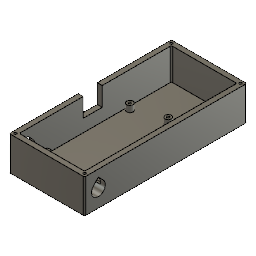
full (Autodesk Fusion 360 design; units mm, degrees)
Autodesk Fusion 360 part; units mm, degrees
sketch "Sketch2" plane through (0, 0, 0) normal (0, 1, 0) x (1, 0, 0)
  line L0 (25, -35.5) -> (-25, -35.5)
  line L1 (-25, -35.5) -> (-25, 35.5)
  line L2 (-25, 35.5) -> (25, 35.5)
  line L3 (25, 35.5) -> (25, -35.5)
  line L4 (25, -35.5) -> (-25, 35.5) construction
  line L5 (-25, -35.5) -> (25, 35.5) construction
  circle A0 centre (-23, -33.5) radius 1
  circle A1 centre (23, -33.5) radius 1
  circle A2 centre (-23, 32.5) radius 1
  circle A3 centre (23, 32.5) radius 1
  line L6 (-25, -1.5) -> (-15, -1.5)
  line L7 (-15, -1.5) -> (-15, 13.5)
  line L8 (-15, 13.5) -> (-25, 13.5)
  line L9 (-25, 13.5) -> (-25, -1.5)
  line L10 (25, 67.5) -> (-21, 67.5)
  line L11 (-21, 67.5) -> (-21, 41.5)
  line L12 (-21, 41.5) -> (25, 41.5)
  line L13 (25, 41.5) -> (25, 67.5)
  line L14 (25, -51.5) -> (7, -51.5)
  line L15 (7, -51.5) -> (7, -41.5)
  line L16 (7, -41.5) -> (25, -41.5)
  line L17 (25, -41.5) -> (25, -51.5)
  line L18 (0, 0) -> (0, -35.5) construction
  line L19 (-25, -41.5) -> (-25, -51.5)
  line L20 (-25, -51.5) -> (-7, -51.5)
  line L21 (-7, -41.5) -> (-25, -41.5)
  line L22 (-7, -51.5) -> (-7, -41.5)
  dimension "d15" = 71
  dimension "d16" = 50
  dimension "d17" = 2
  dimension "d18" = 2
  dimension "d19" = 46
  dimension "d20" = 2
  dimension "d21" = 2
  dimension "d22" = 2
  dimension "d23" = 2
  dimension "d24" = 46
  dimension "d25" = 66
  dimension "d35" = 15
  dimension "d36" = 10
  dimension "d37" = 34
  dimension "d40" = 46
  dimension "d41" = 26
  dimension "d42" = 6
  dimension "d43" = 18
  dimension "d44" = 10
  dimension "d45" = 6
  measures "d17" diameter of A0
  measures "d18" diameter of A1
  measures "d22" diameter of A2
  measures "d37" distance of L0 L6
  measures "d42" distance of L2 L12
  measures "d43" distance of L18.start
  measures "d45" distance of L0 L16
extrude "Extrude2" add sketch "Sketch2" along normal blind 2 contours L0 L1 L2 L3 L6 L7 L8 | L1 L6 L7 L8 L9 makes body 1
extrude "Extrude5" add sketch "Sketch2" along normal blind 18 contours L1 L6 L7 L8 L9 bodies 1
extrude "Extrude7" add sketch "Sketch2" along normal blind 17 separate body contours L10 L11 L12 L13 makes body 2
sketch "Sketch6" plane through (0, 0, 0) normal (0, 1, 0) x (1, 0, 0)
  line L0 (25, 67.5) -> (-25, 67.5)
  line L1 (-25, 67.5) -> (-25, -51.5)
  line L2 (-25, -51.5) -> (25, -51.5)
  line L3 (25, -51.5) -> (25, 67.5)
  line L4 (-30, 72.5) -> (-30, -56.5)
  line L5 (-30, -56.5) -> (30, -56.5)
  line L6 (30, -56.5) -> (30, 72.5)
  line L7 (30, 72.5) -> (-30, 72.5)
  line L8 (-21, 41.5) -> (25, 41.5)
  circle A0 centre (2, 38.0148) radius 2.5
  line L9 (-25, -35.5) -> (-25, 35.5)
  line L10 (-25, 35.5) -> (25, 35.5)
  line L11 (25, 35.5) -> (25, -35.5)
  line L12 (25, -35.5) -> (-25, -35.5)
  circle A1 centre (23, -33.5) radius 1
  circle A2 centre (-23, -33.5) radius 1
  circle A3 centre (-23, 32.5) radius 1
  circle A4 centre (23, 32.5) radius 1
  circle A5 centre (-23, 32.5) radius 2.5
  circle A6 centre (23, 32.5) radius 2.5
  circle A7 centre (23, -33.5) radius 2.5
  circle A8 centre (-23, -33.5) radius 2.5
  line L13 (26, -52.5) -> (26, 68.5)
  line L14 (26, 68.5) -> (-26, 68.5)
  line L15 (-26, 68.5) -> (-26, -52.5)
  line L16 (-26, -52.5) -> (26, -52.5)
  dimension "d53" = 5
  dimension "d60" = 5
  dimension "d66" = 5
  dimension "d67" = 5
  dimension "d68" = 5
  dimension "d69" = 5
  dimension "d101" = 1
  measures "d60" diameter of A0
  measures "d66" diameter of A5
  measures "d67" diameter of A6
  measures "d68" diameter of A7
  measures "d69" diameter of A8
extrude "Extrude9" add sketch "Sketch6" along normal blind 25 separate body contours L4 L5 L6 L7 makes body 3
extrude "Extrude10" add sketch "Sketch6" against normal blind 2 contours L0 L1 L3 L10 | L1 L3 L9 L10 L11 L12 A5 A6 A7 A8 | L1 L9 A5 | L1 L9 A5 | L3 L11 A6 | L3 L11 A6 | L1 L9 L12 A8 | L1 L9 A8 | L3 L11 A7 | L3 L11 L12 A7 | L1 L9 L12 A8 | L3 L11 L12 A7 | L1 L2 L3 L12 A7 A8 | L12 A7 | L12 A8 | L4 L5 L6 L7 | A0 | A1 | A2 | A3 | A4 | L13 L14 L15 L16 bodies 3
extrude "Extrude11" add sketch "Sketch6" along normal blind 5 contours A0 bodies 3
sketch "Sketch7" plane through (0, 5, 0) normal (0, 1, 0) x (-1, 0, 0)
  circle A0 centre (-2, -38.0148) radius 2.5
  circle A1 centre (-2, -38.0148) radius 1
  dimension "d63" = 2
  measures "d63" diameter of A1
extrude "Extrude12" cut sketch "Sketch7" against normal blind 6 contours A1 bodies 3
extrude "Extrude13" add sketch "Sketch6" along normal blind 5 contours L1 L9 A5 | L1 L9 A5 | L3 L11 A6 | L3 L11 A6 | L1 L9 L12 A8 | L1 L9 A8 | L3 L11 A7 | L3 L11 L12 A7 | L12 A7 | L12 A8 picked at (-22.9751, -35.1657) picked at (23.0249, -35.1657) bodies 3
sketch "Sketch8" plane through (-30, 0, 0) normal (-1, 0, 0) x (0, 0, 1)
  line L0 (56.5, -2) -> (56.5, 25)
  line L1 (56.5, 25) -> (-72.5, 25)
  line L2 (-72.5, 25) -> (-72.5, -2)
  line L3 (-72.5, -2) -> (56.5, -2)
  line L4 (1.5, 2) -> (-13.5, 2)
  line L5 (-13.5, 2) -> (-13.5, 18)
  line L6 (-13.5, 18) -> (1.5, 18)
  line L7 (1.5, 18) -> (1.5, 2)
  line L8 (-13.5, 0) -> (1.5, 0)
  line L9 (1.5, 0) -> (1.5, 10)
  line L10 (1.5, 10) -> (-13.5, 10)
  line L11 (-13.5, 10) -> (-13.5, 0)
  line L12 (-13.5, 10) -> (1.5, 10)
  line L13 (1.5, 10) -> (1.5, 20)
  line L14 (1.5, 20) -> (-13.5, 20)
  line L15 (-13.5, 20) -> (-13.5, 10)
  line L16 (-13.5, 10) -> (1.5, 10)
  line L17 (1.5, 10) -> (1.5, 25)
  line L18 (1.5, 25) -> (-13.5, 25)
  line L19 (-13.5, 25) -> (-13.5, 10)
  circle A0 centre (45.5, 11.5) radius 5.5
  line L20 (45.5, 11.5) -> (45.5, 19.5)
  line L21 (45.5, 19.5) -> (41.506, 15.2812)
  line L22 (45.5, 19.5) -> (49.494, 15.2813)
  dimension "d72" = 10
  dimension "d73" = 10
  dimension "d76" = 11
  dimension "d77" = 13.5
  dimension "d78" = 11
  dimension "d84" = 8
  measures "d76" diameter of A0
  measures "d78" distance of L0
sketch "Sketch12" plane through (0, 0, 0) normal (0, 1, 0) x (-1, 0, 0)
  circle A0 centre (-2, -38.0148) radius 2.5
  line L0 (26, 52.5) -> (-26, 52.5)
  line L1 (-26, 52.5) -> (-26, 38.5)
  line L2 (-26, 38.5) -> (26, 38.5)
  line L3 (26, 38.5) -> (26, 52.5)
  line L4 (-11, 52.5) -> (11, 52.5)
  line L5 (11, 52.5) -> (11, 38.5)
  line L6 (11, 38.5) -> (-11, 38.5)
  line L7 (-11, 38.5) -> (-11, 52.5)
  circle A1 centre (23, -32.5) radius 2.5
  circle A2 centre (23, 33.5) radius 2.5
  line L8 (-26, 52.5) -> (-26, -68.5)
  line L9 (-26, -68.5) -> (26, -68.5)
  line L10 (26, -68.5) -> (26, 52.5)
  line L11 (26, 52.5) -> (-26, 52.5)
  circle A3 centre (-23, -32.5) radius 2.5
  circle A4 centre (-23, 33.5) radius 2.5
  circle A5 centre (0, 48.5) radius 1
  circle A6 centre (0, 42.5) radius 1
  line L12 (2.5, 42.5) -> (2.5, 48.5)
  arc A7 (2.5, 48.5) -> (-2.5, 48.5) centre (0, 48.5) ccw
  line L13 (-2.5, 48.5) -> (-2.5, 42.5)
  arc A8 (-2.5, 42.5) -> (2.5, 42.5) centre (0, 42.5) ccw
  line L14 (0, 42.5) -> (0, 48.5) construction
  dimension "d96" = 14
  dimension "d99" = 15
  dimension "d100" = 15
  dimension "d103" = 2
  dimension "d104" = 2
  dimension "d105" = 4
  dimension "d106" = 4
  dimension "d107" = 5
  measures "d99" distance of L1 L7
  measures "d100" distance of L3 L5
  measures "d103" diameter of A5
  measures "d104" diameter of A6
  measures "d105" distance of L6 origin
  measures "d107" diameter of A7
extrude "Extrude19" add sketch "Sketch12" along normal blind 10 contours L0 L2 L3 L5 L10 L11 | L0 L1 L2 L7 L8 L11 bodies 3
extrude "Extrude14" cut sketch "Sketch8" against normal blind 5 contours L1 L14 L17 L18 L19 | L6 L13 L14 L15 L17 L19 | L5 L6 L7 L10 L12 L13 L15 L16 L17 L19 bodies 3
extrude "Extrude16" cut sketch "Sketch8" against normal blind 60 contours A0 | A0 L20 L22 | A0 L20 L21 bodies 3
extrude "Extrude20" add sketch "Sketch12" along normal blind 5 contours L12 A7 L13 A8 bodies 3
sketch "Sketch10" plane through (0, 25, 0) normal (0, 1, 0) x (-1, 0, 0)
  line L0 (30, -13.5) -> (26, -13.5)
  line L1 (26, 1.5) -> (30, 1.5)
  line L2 (30, 1.5) -> (30, 56.5)
  line L3 (30, 56.5) -> (-30, 56.5)
  line L4 (-30, 56.5) -> (-30, -72.5)
  line L5 (-30, -72.5) -> (30, -72.5)
  line L6 (30, -72.5) -> (30, -13.5)
  line L7 (30, -72.5) -> (-30, -72.5)
  line L8 (-30, -72.5) -> (-30, 56.5)
  line L9 (-30, 56.5) -> (30, 56.5)
  line L10 (30, 56.5) -> (30, -72.5)
  circle A0 centre (27.5, 54) radius 1
  circle A1 centre (-27.5, 54) radius 1
  line L11 (-30, -8) -> (30, -8) construction
  circle A2 centre (27.5, -70) radius 1
  circle A3 centre (-27.5, -70) radius 1
  line L12 (26, -13.5) -> (26, -68.5)
  line L13 (26, -68.5) -> (-26, -68.5)
  line L14 (-26, -68.5) -> (-26, 52.5)
  line L15 (-26, 52.5) -> (26, 52.5)
  line L16 (26, 52.5) -> (26, 1.5)
  dimension "d87" = 2
  dimension "d88" = 2.5
  dimension "d89" = 2.5
  dimension "d90" = 2
  dimension "d92" = 2.5
  measures "d87" diameter of A0
  measures "d90" diameter of A1
extrude "Extrude18" cut sketch "Sketch10" against normal blind 10 contours A0 | A1 | A2 | A3 bodies 3
sketch "Sketch14" plane through (0, 5, 0) normal (0, 1, 0) x (-1, 0, 0)
  circle A0 centre (0, 48.5) radius 1
  circle A1 centre (0, 42.5) radius 1
  arc A2 (-2.5, 42.5) -> (2.5, 42.5) centre (0, 42.5) ccw
  line L0 (2.5, 42.5) -> (2.5, 48.5)
  arc A3 (2.5, 48.5) -> (-2.5, 48.5) centre (0, 48.5) ccw
  line L1 (-2.5, 48.5) -> (-2.5, 42.5)
  circle A4 centre (0, 42.5) radius 1.5
  circle A5 centre (0, 48.5) radius 1.5
  dimension "d110" = 3
  dimension "d111" = 3
  measures "d110" diameter of A4
  measures "d111" diameter of A5
extrude "Extrude21" add sketch "Sketch14" along normal blind 5 separate body contours A2 L0 A3 L1 makes body 4
sketch "Sketch15" plane through (0, 10, 0) normal (0, 1, 0) x (-1, 0, 0)
  circle A0 centre (0, 48.5) radius 1.5
  circle A1 centre (0, 42.5) radius 1.5
  line L0 (-2.5, 48.5) -> (-2.5, 42.5)
  arc A2 (-2.5, 42.5) -> (2.5, 42.5) centre (0, 42.5) ccw
  line L1 (2.5, 42.5) -> (2.5, 48.5)
  arc A3 (2.5, 48.5) -> (-2.5, 48.5) centre (0, 48.5) ccw
  line L2 (-22.5, 50.5) -> (22.5, 50.5)
  line L3 (22.5, 50.5) -> (22.5, 39.5)
  line L4 (22.5, 39.5) -> (-22.5, 39.5)
  line L5 (-22.5, 39.5) -> (-22.5, 50.5)
  line L6 (-22.5, 50.5) -> (22.5, 39.5) construction
  line L7 (22.5, 50.5) -> (-22.5, 39.5) construction
  dimension "d114" = 45
extrude "Extrude22" add sketch "Sketch15" along normal blind 3 separate body contours L0 A2 L1 A3 L2 | L0 A2 L1 A3 L2 L3 L4 L5 makes body 5
combine "Combine1" operation add target body 5 tool bodies 4
sketch "Sketch16" plane through (0, 25, 0) normal (0, 1, 0) x (-1, 0, 0)
  line L0 (30, 56.5) -> (-30, 56.5)
  line L1 (-30, 56.5) -> (-30, -72.5)
  line L2 (-30, -72.5) -> (30, -72.5)
  line L3 (30, -72.5) -> (30, -13.5)
  line L4 (30, -13.5) -> (26, -13.5)
  line L5 (26, -13.5) -> (26, -68.5)
  line L6 (26, -68.5) -> (-26, -68.5)
  line L7 (-26, -68.5) -> (-26, 52.5)
  line L8 (-26, 52.5) -> (26, 52.5)
  line L9 (26, 1.5) -> (30, 1.5)
  line L10 (30, 1.5) -> (30, 56.5)
  circle A0 centre (-27.5, -70) radius 1
  circle A1 centre (27.5, 54) radius 1
  circle A2 centre (27.5, -70) radius 1
  circle A3 centre (-27.5, 54) radius 1
  line L11 (30, -13.5) -> (26, -13.5)
  line L12 (26, -13.5) -> (26, 1.5)
  line L13 (26, 1.5) -> (30, 1.5)
  line L14 (30, 1.5) -> (30, -13.5)
  line L15 (26, 52.5) -> (26, 1.5)
  line L16 (24, -13.5) -> (24, -66.5)
  line L17 (24, -66.5) -> (-24, -66.5)
  line L18 (-24, -66.5) -> (-24, 50.5)
  line L19 (-24, 50.5) -> (24, 50.5)
  line L20 (24, 50.5) -> (24, 1.5)
  line L21 (24, -13.5) -> (24, 1.5)
  dimension "d119" = 2
  measures "d119" distance of L5
extrude "Extrude23" add sketch "Sketch16" along normal blind 4 separate body makes body 6
sketch "Sketch17" plane through (0, 0, -72.5) normal (0, 0, -1) x (-1, 0, 0)
  line L0 (-30, 25) -> (30, 25)
  line L1 (30, 25) -> (30, 29)
  line L2 (30, 29) -> (-30, 29)
  line L3 (-30, 29) -> (-30, 25)
  line L4 (0, 29) -> (0, 24.5) construction
  line L5 (-24.3507, 29) -> (-25.2274, 26.8576)
  line L6 (24.3507, 29) -> (25.2274, 26.8576)
  line L7 (-30.2144, 26.8576) -> (29.7856, 26.8576) construction
  line L8 (-24.3507, 29) -> (24.3507, 29)
  line L9 (-25.2274, 26.8576) -> (25.2274, 26.8576)
  line L10 (-25.0039, 27.0076) -> (25.0039, 27.0076)
  line L11 (24.25, 28.85) -> (25.0039, 27.0076)
  line L12 (-24.25, 28.85) -> (24.25, 28.85)
  line L13 (-24.25, 28.85) -> (-25.0039, 27.0076)
  dimension "d128" = 0.15
extrude "Extrude25" cut sketch "Sketch17" against normal blind 122 contours L2 L5 L6 L8 L9 | L10 L11 L12 L13 bodies 6
extrude "Extrude26" add sketch "Sketch17" against normal blind 121.5 separate body contours L10 L11 L12 L13 makes body 7
fillet "Fillet2" radius 1 4 edges at (-30, 11.5, -72.5) (30, 11.5, -72.5) (30, 11.5, 56.5) (-30, 11.5, 56.5) on bodies 3
fillet "Fillet3" radius 1 4 edges at (-26, 17.5, 52.5) (26, 17.5, 52.5) (26, 12.5, -68.5) (-26, 12.5, -68.5) on bodies 3
hidden bodies 1 2 5 6 7
named bodies: "board", "battery", "case", "motor_mount", "mount", "lid", "clamp"
